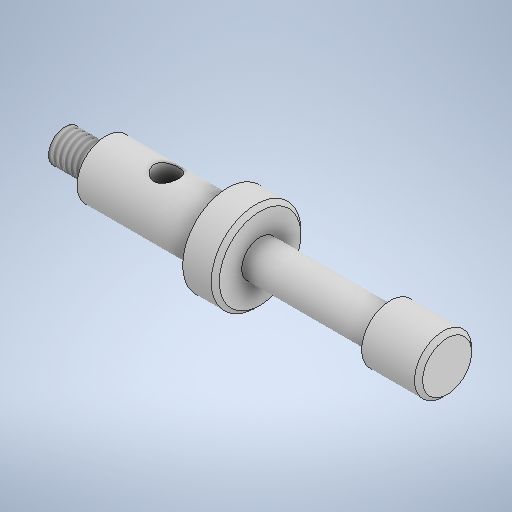
# Autodesk Inventor part: 151
Saved by Autodesk Inventor 2025.1 (Build 291241000, 241)
## iProperties
Created: 2024-08-05
Part Number: 151
Material: Generisch
Document SubType Name: Modeling
Designer: ffogue
Density: 1 g/cm^3
Appearance: Vorgabe
Author: ffogue
Autodesk Inventor part; units mm, degrees
ref_plane "YZ Plane" through (0, 0, 0) normal (1, 0, 0) x (0, 1, 0)
ref_plane "XZ Plane" through (0, 0, 0) normal (0, 1, 0) x (-1, 0, 0)
sketch "Sketch1" plane through (0, 0, 0) normal (0, 0, 1) x (1, 0, 0)
  line L0 (0, 0) -> (0, 2)
  line L1 (0, 2) -> (5, 2)
  line L2 (5, 2) -> (5, 3.5)
  line L3 (5, 3.5) -> (20, 3.5)
  line L4 (20, 3.5) -> (20, 5.5)
  line L5 (20, 5.5) -> (21.4643, 5.5)
  line L6 (21.4643, 5.5) -> (21.4643, 5.5)
  line L7 (21.4643, 5.5) -> (24, 5.5)
  line L8 (24, 5.5) -> (24, 2.25)
  line L9 (24, 2.25) -> (40, 2.25)
  line L10 (40, 2.25) -> (40, 3.5)
  line L11 (40, 3.5) -> (47, 3.5)
  line L12 (47, 3.5) -> (47, 0)
  line L13 (47, 0) -> (0, 0)
  dimension "d0" = 4
  dimension "d1" = 7
  dimension "d2" = 5
  dimension "d3" = 15
  dimension "d4" = 47
  dimension "d5" = 7
  dimension "d6" = 16
  dimension "d7" = 4.5
  dimension "d8" = 4
  dimension "d10" = 11
  constraints: 28 end point, 12 perpendicular, 2 point on line, 1 coincident, 1 vertical
  measures "d0" diameter of L1 L13
  measures "d1" diameter of L3 L13
  measures "d2" distance of L0.end L1.end
  measures "d3" distance of L2.end L3.end
  measures "d4" distance between parallel lines of L12 L0
  measures "d5" distance of L10.end L11.end
  measures "d6" distance of L8.end L9.end
  measures "d7" diameter of L9 L13
  measures "d8" distance between parallel lines of L8 L4
  measures "d10" diameter of L7 L13
revolve "Revolution1" add sketch "Sketch1" angle 360 about axis through (47, 0, 0) along (-1, 0, 0)
thread "Thread1" size "M4x0.7" class "6g" standard "ISO Metric profile" length 10
chamfer "Chamfer1" distance 0.5 angle 45 2 edges at (24, -5.5, 0) (47, -3.5, 0)
ref_plane "Work Plane1" through (0, 0, 3.5) normal (0, 0, 1) x (1, 0, 0)
sketch "Sketch2" plane through (0, 0, 3.5) normal (0, 0, 1) x (1, 0, 0)
  line L0 (5, 3.5) -> (5, -3.5) projected
  point P0 (0, 0)
  point P1 (12.5, 0)
  dimension "d18" = 7.5
  constraints: 1 horizontal alignment
  measures "d18" distance from line of point (12.5, 0) L0
hole "Hole1" at (12.5, 0, 3.5) direction (0, 0, -1) diameter 3 end through all
sketch "Sketch4" plane through (0, 0, 0) normal (0, 0, 1) x (1, 0, 0)
  line L0 (44.893, 3.5) -> (42.8722, 0)
  line L1 (46.5, 3.5) -> (44.893, 3.5)
  line L2 (47, 3) -> (47, -3) projected
  line L3 (46.5, 3.5) -> (40, 3.5) projected
  line L4 (46.5, -3.5) -> (46.5, 3.5) projected
  line L5 (46.5, 3.5) -> (44.4793, 0)
  line L6 (44.4793, 0) -> (42.8722, 0)
  point P0 (0, 0)
  point P1 (44.4443, 0)
  point P2 (47, 0)
  point P3 (46.5, 0)
  dimension "d38" = 30
  constraints: 8 end point, 4 horizontal alignment, 2 midpoint, 1 parallel, 1 point on line
  measures "d38" angle of L4 L5
revolve "Revolution3" cut sketch "Sketch4" angle 360 about axis through (44.893, 3.5, 0) along (0.5, 0.8660254, 0)
body "Solid1"
